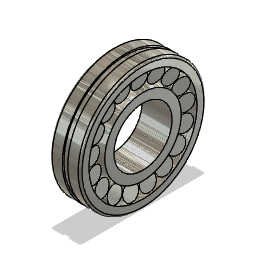
BearingSim v16 (Autodesk Fusion 360 design; units mm, degrees)
Autodesk Fusion 360 part; units mm, degrees
sketch "Sketch1" plane through (0, 0, 0) normal (0, 0, 1) x (1, 0, 0)
  line L0 (0, 0) -> (0, 42) construction
  line L1 (-15.5, 0) -> (15.5, 0) construction
  line L2 (-15.5, 30) -> (15.5, 30)
  arc A0 (15.5, 55.890518) -> (-15.5, 55.890518) centre (0, 0) ccw
  line L3 (-15.5, 30) -> (-15.5, 39.499977)
  line L4 (15.5, 39.499977) -> (15.5, 30)
  arc A1 (-15.5, 39.499977) -> (0, 42) centre (-16.900581, 97.483064) ccw
  arc A2 (0, 42) -> (15.5, 39.499977) centre (16.900581, 97.483064) ccw
  line L5 (15.5, 39.499977) -> (15.5, 57.991327) construction
  line L6 (-15.5, 39.499977) -> (-15.5, 57.991327) construction
  line L7 (-15.5, 55.890518) -> (-15.5, 63)
  line L8 (-13.5, 65) -> (-2.75, 65)
  line L9 (-2.75, 65) -> (-2.75, 63.5)
  line L10 (-2.75, 63.5) -> (2.75, 63.5)
  line L11 (2.75, 63.5) -> (2.75, 65)
  line L12 (2.75, 65) -> (13.5, 65)
  line L13 (15.5, 63) -> (15.5, 55.890518)
  line L14 (-13.077087, 56.506547) -> (-10.144997, 39.877838) construction
  line L15 (-5.176201, 57.768564) -> (-2.282139, 41.35552) construction
  line L16 (0, 0) -> (-10.071594, 57.11885) construction
  line L17 (-11.611042, 48.192192) -> (-3.72917, 49.562042) construction
  arc A3 (-13.5, 65) -> (-15.5, 63) centre (-13.5, 63) ccw
  arc A4 (15.5, 63) -> (13.5, 65) centre (13.5, 63) ccw
  line L18 (23.547757, 26) -> (-28.717196, 26) construction
  dimension "d1" = 42
  dimension "d2" = 31
  dimension "d3" = 31
  dimension "d4" = 30
  dimension "d5" = 58
  dimension "d6" = 58
  dimension "d7" = 65
  dimension "d8" = 65
  dimension "d9" = 1.5
  dimension "d10" = 5.5
  dimension "d11" = 2.5
  dimension "d12" = 8
  dimension "d13" = 10
  dimension "d14" = 2
  dimension "d21" = 4
  constraint coincident L0.start A0.centre
  constraint vertical L0
  constraint horizontal L1
  constraint symmetric L0 L1.start L1.end
  constraint horizontal L2
  constraint symmetric L0 L2.start L2.end
  constraint perpendicular L2 L3
  constraint perpendicular L2 L4
  constraint symmetric A1.end L0 A2.start
  constraint symmetric L0 A1 A2
  constraint parallel L4 L5
  constraint parallel L6 L7
  constraint perpendicular L6 L8
  constraint perpendicular L8 L9
  constraint perpendicular L6 L10
  constraint perpendicular L10 L11
  constraint perpendicular L5 L12
  constraint perpendicular L12 L13
  constraint symmetric L0 L9 L11
  constraint parallel L14 L15
  constraint parallel L15 L16
  constraint tangent L7 A3
  constraint tangent L8 A3
  constraint tangent L12 A4
  constraint tangent L13 A4
  constraint equal A3 A4
  constraint perpendicular L0 L18
  measures "d1" distance of L0.start L0.end
  measures "d2" distance of L1.start L1.end
  measures "d3" distance of L2.start L2.end
  measures "d4" distance of L1 L2
  measures "d5" radius of A0
  measures "d6" radius of A1
  measures "d7" distance of L1 L8
  measures "d8" distance of L1 L12
  measures "d9" distance of L10 L12
  measures "d10" distance of L9 L11
  measures "d12" distance of L14 L15
  measures "d13" angle of L0 L16
  measures "d14" radius of A3
  measures "d21" distance of L2 L18
revolve "Revolve1" add sketch "Sketch1" angle 360 about axis through (-15.5, 0, 0) along (1, 0, 0) contours L2 L3 L4 A1 A2 | A0 L7 L8 L9 L10 L11 L12 L13 A3 A4 picked at (1.69469, 33.566509) picked at (8.023815, 61.99007) makes body 1 at (1.743148, -28.9869, -50.206783) makes body 2 at (-5.166667, 29.962708, -1.495377)
sketch "Sketch2" plane through (0, 0, 0) normal (0, 0, 1) x (1, 0, 0)
  arc A0 (15.5, 55.890518) -> (-15.5, 55.890518) centre (0, 0) ccw
  line L0 (-5.176201, 57.768564) -> (-2.282139, 41.35552)
  line L1 (-11.611042, 48.192192) -> (-3.72917, 49.562042)
  line L2 (-13.077087, 56.506547) -> (-10.144997, 39.877838)
  line L3 (-13.077087, 56.506547) -> (-11.611042, 48.192192)
  line L4 (-11.611042, 48.192192) -> (-3.72917, 49.562042)
  line L5 (-3.72917, 49.562042) -> (-5.176201, 57.768564)
  arc A1 (-5.176201, 57.768564) -> (-13.077087, 56.506547) centre (0, 0) ccw
revolve "Revolve2" add sketch "Sketch2" angle 360 about axis through (-11.611042, 48.192192, 0) along (0.98523096, 0.17123071, 0) separate body contours A0 L0 L1 L2 L3 L4 L5 A1 picked at (-7.722826, 51.741172) makes body 3
mirror "Mirror1" about plane through (0, 0, 0) normal (1, 0, 0) of bodies 3 makes body 4
pattern_circular "C-Pattern1" count 17 over 360 about axis through (16.900581, 0, 0) along (1, 0, 0) of bodies 3 4 makes body 5 at (-7.799434, 54.041687, 19.131275) makes body 6 at (-7.799434, 43.481358, 37.361492) makes body 7 at (-7.799434, 27.048631, 50.545832) makes body 8 at (-7.799434, 6.962837, 56.903677) makes body 9 at (-7.799434, -14.063327, 55.576366) makes body 10 at (7.799434, 54.041687, 19.131275) makes body 11 at (7.799434, 43.481358, 37.361492) makes body 12 at (7.799434, 27.048631, 50.545832) makes body 13 at (7.799434, 6.962837, 56.903677) makes body 14 at (7.799434, -14.063327, 55.576366) makes body 15 at (-7.799434, -33.190161, 46.743158) makes body 16 at (-7.799434, -47.834479, 31.597028) makes body 17 at (-7.799434, -56.018487, 12.183544) makes body 18 at (-7.799434, -56.636887, -8.875395) makes body 19 at (-7.799434, -49.606162, -28.735663) makes body 20 at (-7.799434, -35.875849, -44.71502) makes body 21 at (-7.799434, -17.300305, -54.655366) makes body 22 at (-7.799434, 3.611742, -57.214202) makes body 23 at (-7.799434, 24.036002, -52.045943) makes body 24 at (-7.799434, 41.214068, -39.848591) makes body 25 at (-7.799434, 52.825945, -22.269466) makes body 26 at (7.799434, -33.190161, 46.743158) makes body 27 at (7.799434, -47.834479, 31.597028) makes body 28 at (7.799434, -56.018487, 12.183544) makes body 29 at (7.799434, -56.636887, -8.875395) makes body 30 at (7.799434, -49.606162, -28.735663) makes body 31 at (7.799434, -35.875849, -44.71502) makes body 32 at (7.799434, -17.300305, -54.655366) makes body 33 at (7.799434, 3.611742, -57.214202) makes body 34 at (7.799434, 24.036002, -52.045943) makes body 35 at (7.799434, 41.214068, -39.848591) makes body 36 at (7.799434, 52.825945, -22.269466)
named bodies: "Outer ring", "Inner raceway", "Bearing1", "Bearing2", "Bearing3", "Bearing4", "Bearing5", "Bearing6", "Bearing7", "Bearing8", "Bearing9", "Bearing10", "Bearing11", "Bearing12", "Bearing1 (1)", "Bearing1 (2)", "Bearing1 (3)", "Bearing1 (4)", "Bearing1 (5)", "Bearing1 (6)", "Bearing1 (7)", "Bearing1 (8)", "Bearing1 (9)", "Bearing1 (10)", "Bearing1 (11)", "Bearing2 (1)", "Bearing2 (2)", "Bearing2 (3)", "Bearing2 (4)", "Bearing2 (5)", "Bearing2 (6)", "Bearing2 (7)", "Bearing2 (8)", "Bearing2 (9)", "Bearing2 (10)", "Bearing2 (11)"
